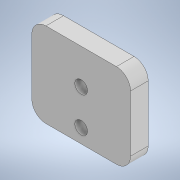
# Autodesk Inventor part: hold gt2
Saved by Autodesk Inventor 2020 (Build 240168000, 168)
## iProperties
Created: 2026-07-08
Part Number: hold gt2
Material: Generic
Document SubType Name: Modeling
Designer: drago
Density: 1 g/cm^3
Appearance: Default
Author: drago
Autodesk Inventor part; units mm, degrees
ref_plane "YZ Plane" through (0, 0, 0) normal (1, 0, 0) x (0, 1, 0)
ref_plane "XZ Plane" through (0, 0, 0) normal (0, 1, 0) x (-1, 0, 0)
ref_plane "XY Plane" through (0, 0, 0) normal (0, 0, 1) x (1, 0, 0)
sketch "Sketch1" plane through (0, 0, 0) normal (0, 0, 1) x (1, 0, 0)
  arc A0 (7, 17.5) -> (5, 19.5) centre (5, 17.5) ccw
  line L0 (5, 19.5) -> (-5, 19.5)
  arc A1 (-5, 19.5) -> (-7, 17.5) centre (-5, 17.5) ccw
  line L1 (-7, 17.5) -> (-7, 9.5)
  line L2 (7, 9.5) -> (7, 17.5)
  circle A2 centre (0, 14.5) radius 0.9
  circle A3 centre (0, 9.5) radius 0.9
  line L3 (7, 17.5) -> (7, 9.5)
  line L4 (5, 7.5) -> (-5, 7.5)
  arc A4 (5, 7.5) -> (7, 9.5) centre (5, 9.5) ccw
  arc A5 (-7, 9.5) -> (-5, 7.5) centre (-5, 9.5) ccw
  point P0 (0, 0)
  point P1 (0, 0)
  constraints: 10 end point, 8 point on circle, 6 centre point, 4 tangent, 1 equal radius, 1 perpendicular
extrude "Extrusion1" add sketch "Sketch1" along normal blind 2.5
body "Solid1"
